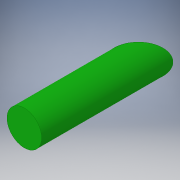
# Autodesk Inventor part: Pool Noodle
Saved by Autodesk Inventor 2017 (Build 210142000, 142)
## iProperties
Created: 2017-02-12
Part Number: Pool Noodle
Material: Generic
Document SubType Name: Modeling
Designer: kingb
Density: 1 g/cm^3
Appearance: Dark Green
Author: kingb
Autodesk Inventor part; units mm, degrees
ref_plane "XZ Plane" through (0, 0, 0) normal (0, 1, 0) x (-1, 0, 0)
ref_plane "XY Plane" through (0, 0, 0) normal (0, 0, 1) x (1, 0, 0)
sketch "Sketch1" plane through (0, 0, 0) normal (0, 0, 1) x (1, 0, 0)
  circle A0 centre (0, 0) radius 31.75
  dimension "d0" = 63.5
  constraints: 1 centre point, 1 coincident
  measures "d0" diameter of A0
ref_plane "Work Plane1" through (-31.75, 0, 0) normal (1, 0, 0) x (0, 1, 0)
extrude "Extrusion2" add sketch "Sketch1" against normal blind 241.3
sketch "Sketch3" plane through (0, 0, 0) normal (0, 1, 0) x (-1, 0, 0)
  line L0 (-31.75, -241.3) -> (31.75, -241.3) projected
  line L1 (-31.75, -241.3) -> (31.75, -241.3)
  line L2 (31.75, -241.3) -> (31.75, -177.8)
  line L3 (31.75, -177.8) -> (-31.75, -177.8)
  line L4 (-31.75, -177.8) -> (-31.75, -241.3)
  line L5 (-31.75, -241.3) -> (31.75, -177.8)
  point P0 (0, 0)
  dimension "d7" = 63.5
  dimension "d8" = 63.5
  constraints: 10 end point, 2 parallel, 1 horizontal, 1 perpendicular
  measures "d7" distance of L3.end L2.end
  measures "d8" distance of L2.end L1.end
extrude "Extrusion3" cut sketch "Sketch3" along normal mid plane 63.5 contours L5 L2 L0
body "Solid2"
